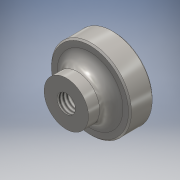
# Autodesk Inventor part: Bed Thumb Screw
Saved by Autodesk Inventor 2016 (Build 200138000, 138)
## iProperties
Created: 2017-04-14
Part Number: Bed Thumb Screw
Material: Stainless Steel
Document SubType Name: Modeling
Designer: Scott
Density: 8 g/cm^3
Appearance: Semi-Polished
Author: Scott
Autodesk Inventor part; units mm, degrees
ref_plane "YZ Plane" through (0, 0, 0) normal (1, 0, 0) x (0, 1, 0)
ref_plane "XZ Plane" through (0, 0, 0) normal (0, 1, 0) x (-1, 0, 0)
ref_plane "XY Plane" through (0, 0, 0) normal (0, 0, 1) x (1, 0, 0)
sketch "Sketch1" plane through (0, 0, 0) normal (0, 0, 1) x (1, 0, 0)
  line L0 (0, 0) -> (0, 12.3467)
  line L1 (0, 0) -> (3, 0)
  line L2 (3, 0) -> (3, 1.5)
  line L3 (3, 1.5) -> (2.85, 1.5)
  line L4 (2.85, 1.5) -> (2.85, 3.2)
  line L5 (2.85, 3.2) -> (5.4, 3.2)
  line L6 (5.4, 3.2) -> (5.4, 6.4)
  line L7 (5.4, 6.4) -> (0, 6.4)
  line L8 (0, 0) -> (0, 6.4)
  dimension "d1" = 5.7
  dimension "d2" = 6
  dimension "d3" = 10.8
  dimension "d4" = 1.5
  dimension "d6" = 6.4
  dimension "d7" = 3.2
  constraints: 18 end point, 5 perpendicular, 2 vertical, 1 collinear, 1 horizontal, 1 point on line
  measures "d1" diameter of L4 L0
  measures "d2" diameter of L2 L0
  measures "d3" diameter of L6 L0
  measures "d4" distance of L1.end L2.end
  measures "d6" distance between parallel lines of L1 L7
  measures "d7" distance of L5.end L6.end
revolve "Revolution1" add sketch "Sketch1" angle 360 about axis through (0, 0, 0) along (0, 1, 0)
fillet "Fillet1" radius 1.6 1 edges at (-2.85, 3.2, 0)
chamfer "Chamfer1" distance 0.2 angle 45 2 edges at (-5.4, 6.4, 0) (-5.4, 3.2, 0)
hole "Hole1" at (0, 6.4, 0) direction (0, -1, 0) diameter 2.459 end through all thread size "M3x0.5" class "6H" standard "ISO Metric profile"
body "Solid1"
